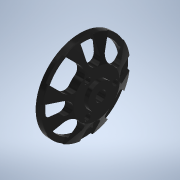
# Autodesk Inventor part: TOP
Saved by Autodesk Inventor 2022 (Build 260153000, 153)
## iProperties
Created: 2022-07-25
Part Number: TOP
Material: Stainless Steel
Document SubType Name: Modeling
Designer: Nathan Cai
Density: 8 g/cm^3
Appearance: Smooth - Black
Author: Nathan Cai
Autodesk Inventor part; units mm, degrees
ref_plane "YZ Plane" through (0, 0, 0) normal (1, 0, 0) x (0, 1, 0)
ref_plane "XZ Plane" through (0, 0, 0) normal (0, 1, 0) x (-1, 0, 0)
ref_plane "XY Plane" through (0, 0, 0) normal (0, 0, 1) x (1, 0, 0)
sketch "Sketch1" plane through (0, 0, 0) normal (0, 0, 1) x (1, 0, 0)
  line L0 (0, 0) -> (3, 0)
  line L1 (3, 0) -> (3, 21) construction
  line L2 (3, 21) -> (0, 21)
  line L3 (0, 21) -> (0, 0) construction
  line L4 (0, 0) -> (8, 0)
  line L5 (8, 0) -> (8, 11)
  line L6 (8, 11) -> (0, 11) construction
  line L7 (0, 11) -> (0, 0) construction
  line L8 (3, 21) -> (8, 11)
  line L9 (8, 0) -> (10, 0)
  line L10 (10, 0) -> (10, 6)
  line L11 (10, 6) -> (8, 6)
  line L12 (8, 6) -> (8, 0)
  line L13 (0, 0) -> (10, 0)
  line L14 (10, 0) -> (10, 2.5)
  line L15 (10, 2.5) -> (-0.3, 2.5)
  line L16 (0, 2.5) -> (0, 0)
  line L17 (8, 11) -> (4, 11) construction
  line L18 (4, 11) -> (4, 0)
  line L19 (4, 0) -> (8, 0)
  line L20 (8, 0) -> (8, 11)
  line L21 (0, 21) -> (3, 21)
  line L22 (3, 21) -> (3, 18.5) construction
  line L23 (3, 18.5) -> (0, 18.5)
  line L24 (0, 18.5) -> (0, 21)
  line L25 (3, 18.5) -> (4, 11)
  line L26 (4, 0) -> (3.25, 0)
  line L27 (3.25, 0) -> (3.25, 7.5)
  line L28 (3.25, 7.5) -> (4, 7.5)
  line L29 (4, 7.5) -> (4, 0)
  line L30 (3.25, 0) -> (-0.3, 0)
  line L31 (-0.3, 0) -> (-0.3, 5.5)
  line L32 (-0.3, 5.5) -> (3.25, 5.5) construction
  line L33 (3.25, 5.5) -> (3.25, 0)
  line L34 (-0.3, 3.75) -> (3.25, 5.5)
  point P0 (8, 2.5)
  dimension "d0" = 3
  dimension "d1" = 21
  dimension "d2" = 8
  dimension "d3" = 11
  dimension "d4" = 2
  dimension "d5" = 6
  dimension "d6" = 2.5
  dimension "d8" = 4
  dimension "d9" = 2.5
  dimension "d10" = 0.75
  dimension "d11" = 7.5
  dimension "d12" = 3.55
  dimension "d13" = 5.5
  dimension "d15" = 3.75
  constraints: 70 end point, 16 parallel, 8 horizontal, 8 perpendicular, 6 point on line
  measures "d0" distance of L2.end L1.end
  measures "d1" distance of L1.end L0.end
  measures "d2" distance of L6.end L5.end
  measures "d3" distance of L5.end L4.end
  measures "d4" distance of L11.end L10.end
  measures "d5" distance of L10.end L9.end
  measures "d6" distance of L14.end L13.end
  measures "d8" distance of L19.end L18.end
  measures "d9" distance of L21.end L22.end
  measures "d10" distance of L27.end L28.end
  measures "d11" distance of L26.end L27.end
  measures "d12" distance of L31.end L32.end
  measures "d13" distance of L30.end L31.end
  measures "d15" distance from line of L30 L34.start
revolve "Revolution1" add sketch "Sketch1" angle 360 about axis through (0, 0, 0) along (1, 0, 0) contours L15 L31 L34 L27 | L27 L28 L18 L15 | L18 L25 L23 L24 L2 L8 L5 L15 | L5 L11 L10 L15
sketch "Sketch2" plane through (8, 0, 0) normal (1, 0, 0) x (0, 0, -1)
  arc A0 (3.125, -14.125) -> (-3.125, -14.125) centre (0, -14.125) ccw
  line L0 (0, 0) -> (0, -14.125) construction
  circle A1 centre (0, 0) radius 2.5 projected
  line L1 (3.125, -14.125) -> (3.125, -20.7662)
  circle A2 centre (0, 0) radius 21 projected
  line L2 (-3.125, -14.125) -> (-3.125, -20.7662)
  line L3 (0, 0) -> (-14.8492, -14.8492)
  circle A3 centre (0, 0) radius 11
  arc A4 (-5.3033, -13.0815) -> (-13.0815, -5.3033) centre (-9.1924, -9.1924) ccw
  line L4 (-5.3033, -13.0815) -> (-10.4418, -18.22)
  line L5 (-13.0815, -5.3033) -> (-18.22, -10.4418)
  arc A5 (14.125, 3.125) -> (14.125, -3.125) centre (14.125, 0) ccw
  line L6 (14.125, 3.125) -> (20.7662, 3.125)
  line L7 (14.125, -3.125) -> (20.7662, -3.125)
  arc A6 (13.0815, -5.3033) -> (5.3033, -13.0815) centre (9.1924, -9.1924) ccw
  line L8 (13.0815, -5.3033) -> (18.22, -10.4418)
  line L9 (5.3033, -13.0815) -> (10.4418, -18.22)
  arc A7 (-3.125, 14.125) -> (3.125, 14.125) centre (0, 14.125) ccw
  line L10 (-3.125, 14.125) -> (-3.125, 20.7662)
  line L11 (3.125, 14.125) -> (3.125, 20.7662)
  arc A8 (5.3033, 13.0815) -> (13.0815, 5.3033) centre (9.1924, 9.1924) ccw
  line L12 (5.3033, 13.0815) -> (10.4418, 18.22)
  line L13 (13.0815, 5.3033) -> (18.22, 10.4418)
  arc A9 (-14.125, -3.125) -> (-14.125, 3.125) centre (-14.125, 0) ccw
  line L14 (-14.125, -3.125) -> (-20.7662, -3.125)
  line L15 (-14.125, 3.125) -> (-20.7662, 3.125)
  arc A10 (-13.0815, 5.3033) -> (-5.3033, 13.0815) centre (-9.1924, 9.1924) ccw
  line L16 (-13.0815, 5.3033) -> (-18.22, 10.4418)
  line L17 (-5.3033, 13.0815) -> (-10.4418, 18.22)
  line L18 (8.6603, 0) -> (-4.3301, -7.5) construction
  line L19 (-4.3301, -7.5) -> (-4.3301, 7.5) construction
  line L20 (-4.3301, 7.5) -> (8.6603, 0) construction
  circle A11 centre (8.6603, 0) radius 1.5
  line L21 (0.2479, 0) -> (8.6603, 0)
  circle A12 centre (-4.3301, 7.5) radius 1.5
  circle A13 centre (-4.3301, -7.5) radius 1.5
  point P0 (14.8492, -14.8492)
  point P1 (14.8492, 14.8492)
  point P2 (-14.8492, 14.8492)
  point P3 (-10.3194, 3.8091)
  point P4 (-3.8091, 10.3194)
  point P5 (-3.8091, -10.3194)
  point P6 (-10.3194, -3.8091)
  point P7 (10.3194, -3.8091)
  point P8 (3.8091, -10.3194)
  point P9 (3.8091, 10.3194)
  point P10 (10.3194, 3.8091)
  dimension "d16" = 6.25
  dimension "d18" = 45
  dimension "d19" = 11
  dimension "d20" = 13
  dimension "d21" = 22
  dimension "d24" = 360
  dimension "d30" = 15
  dimension "d31" = 3
  dimension "d34" = 360
  constraints: 44 end point, 20 point on circle, 12 centre point, 4 tangent, 3 coincident, 2 parallel, 2 point on line, 2 symmetric about line, 2 vertical, 1 horizontal, 83 other
  measures "d16" diameter of A0
  measures "d18" angle of L0 L3
  measures "d19" diameter of A4
  measures "d20" distance of A1.centre A4.centre
  measures "d21" diameter of A3
  measures "d30" distance of L18.end L19.end
  measures "d31" diameter of A11
extrude "Extrusion1" cut sketch "Sketch2" against normal blind 6 contours L1 A2 L2 A0 | A4 L4 A2 L3 A3 | A3 A6 L8 A2 L9 | L3 A2 L5 A4 A3 | A13 A4 | A4 A13 | A5 L6 A2 L7 | A9 L14 A2 L15 | A3 A8 L12 A2 L13 | A10 L16 A2 L17 A3 | A12 A10 | A10 A12 | A7 L10 A2 L11 | A11
fillet "Fillet1" radius 3.175 8 edges at (6, 3.8091, -10.3194) (6, 10.3194, -3.8091) (6, 10.3194, 3.8091) (6, 3.8091, 10.3194) (6, -3.8091, 10.3194) (6, -10.3194, 3.8091) (6, -10.3194, -3.8091) (6, -3.8091, -10.3194)
fillet "Fillet2" radius 0.5 8 edges at (3, 6.9018, -19.8334) (3, 19.8334, -6.9018) (3, 19.8334, 6.9018) (3, -6.9018, -19.8334) (3, -19.8334, -6.9018) (3, -19.8334, 6.9018) (3, -6.9018, 19.8334) (3, 6.9018, 19.8334)
body "Solid1"
